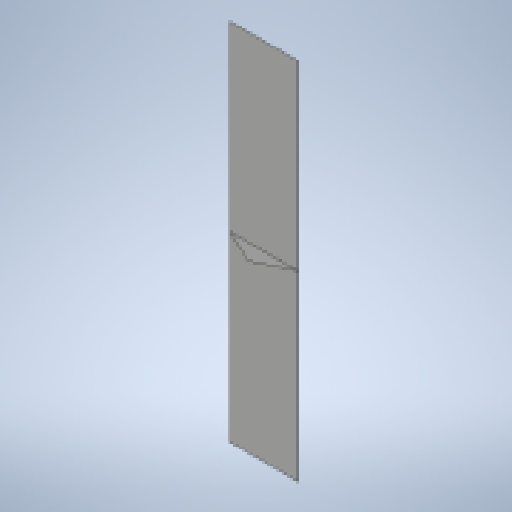
# Autodesk Inventor part: FOVcam
Saved by Autodesk Inventor 2025.1 (Build 291241000, 241)
## iProperties
Created: 2026-04-13
Part Number: FOVcam
Material: Generic
Document SubType Name: Modeling
Designer: User
Density: 1 g/cm^3
Appearance: Default
Author: User
Autodesk Inventor part; units mm, degrees
ref_plane "YZ Plane" through (0, 0, 0) normal (1, 0, 0) x (0, 1, 0)
ref_plane "XZ Plane" through (0, 0, 0) normal (0, 1, 0) x (-1, 0, 0)
ref_plane "XY Plane" through (0, 0, 0) normal (0, 0, 1) x (1, 0, 0)
sketch "Sketch1" plane through (0, 0, 0) normal (0, 1, 0) x (-1, 0, 0)
  line L0 (7, 0) -> (-7, 0) projected
  arc A0 (-5, -3.7812) -> (5, -3.7812) centre (0, 9.3638) ccw
  line L1 (0, -4.7) -> (163.1354, -80.7713)
  line L2 (0, -4.7) -> (180, -4.7) construction
  line L3 (0, -4.7) -> (97.3734, -4.7) construction
  line L4 (0, -4.7) -> (-163.1354, -80.7713)
  line L5 (0, -4.7) -> (180, -4.7) construction
  line L6 (-163.1354, -80.7713) -> (163.1354, -80.7713)
  point P0 (0, 0)
  constraints: 12 end point, 3 horizontal, 3 point on circle, 2 equal length, 1 centre point, 4 other
extrude "Extrusion1" add sketch "Sketch1" along normal blind 0.1
sketch "Sketch3" plane through (163.1354, 0, -80.7713) normal (0, 0, -1) x (-1, 0, 0)
  line L0 (0, 0) -> (326.2708, 0) projected
  line L1 (326.2708, 0) -> (326.2708, 0.1) projected
  line L2 (0, 0.1) -> (326.2708, 0.1) projected
  line L3 (0, 0) -> (0, 0.1) projected
  point P0 (163.1354, 0)
extrude "Extrusion2" add sketch "Sketch3" along normal blind 0.1
sketch "Sketch4" plane through (163.1354, 0, -80.7713) normal (1, 0, 0) x (0, 0, -1)
  line L0 (-76.0713, 0) -> (0, 0) projected
  line L1 (-76.0713, 0) -> (0, -869.4988)
  line L2 (-76.0713, 0) -> (796.7488, 0) construction
  line L3 (-76.0713, 0) -> (0, 869.4988)
  line L4 (-76.0713, 0) -> (796.7488, 0) construction
  line L5 (0, 869.4988) -> (0, -869.4988)
  point P0 (-80.7713, 0)
  dimension "d10" = 85
  dimension "d11" = 85
  constraints: 10 end point, 2 equal length, 2 horizontal, 1 vertical
  measures "d10" angle of L1 L2
  measures "d11" angle of L4 L3
extrude "Extrusion3" add sketch "Sketch4" along normal blind 0.1
sketch "Sketch5" plane through (163.1354, 0, -80.8713) normal (0, 0, -1) x (-1, 0, 0)
  line L0 (0, -869.4988) -> (0, 0) projected
  line L1 (0, 0.1) -> (0, 0) projected
  line L2 (0, 0.1) -> (0, 869.4988) projected
  line L3 (0, 0) -> (326.2708, 0) projected
  line L4 (0, -869.4988) -> (326.2708, -869.4988)
  line L5 (326.2708, -869.4988) -> (326.2708, 869.4988)
  line L6 (326.2708, 869.4988) -> (0, 869.4988)
  line L7 (0, 869.4988) -> (0, -869.4988)
  point P0 (163.1354, 0)
  constraints: 8 end point, 2 parallel, 1 horizontal, 1 perpendicular
extrude "Extrusion4" add sketch "Sketch5" along normal blind 0.1
sketch "Sketch6" plane through (163.2354, 0, -80.7713) normal (1, 0, 0) x (0, 0, -1)
  line L0 (0, -869.4988) -> (0, 0) projected
  line L1 (-76.0713, 0) -> (0, -869.4988) projected
  line L2 (0, 869.4988) -> (-76.0713, 0) projected
  line L3 (0, 0.1) -> (0, 869.4988) projected
  line L4 (0, 0) -> (0, 0.1) projected
  point P0 (-80.7713, 0)
extrude "Extrusion5" cut sketch "Sketch6" against normal blind 0.1
body "Solid1"
